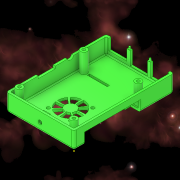
# Autodesk Inventor part: Bodem
Saved by Autodesk Inventor 2017 (Build 210142000, 142)
## iProperties
Created: 2016-12-17
Part Number: Bodem
Material: ABS Plastic
Document SubType Name: Modeling
Designer: bartv
Density: 1.06 g/cm^3
Appearance: Smooth - White
Author: bartv
## iProperties of the stored document Deksel_3DPrint.ipt
Created: 2016-12-19
Part Number: Deksel_3DPrint
Material: Generic
Document SubType Name: Modeling
Designer: bartv
Density: 1 g/cm^3
Appearance: Default
Author: bartv
Autodesk Inventor part; units mm, degrees
ref_plane "YZ Plane" through (0, 0, 0) normal (1, 0, 0) x (0, 1, 0)
ref_plane "XZ Plane" through (0, 0, 0) normal (0, 1, 0) x (-1, 0, 0)
ref_plane "XY Plane" through (0, 0, 0) normal (0, 0, 1) x (1, 0, 0)
sketch "Sketch3" plane through (0, 0, 0) normal (0, 1, 0) x (-1, 0, 0)
  line L0 (0, 0) -> (61, 0)
  line L1 (61, 0) -> (61, -90)
  line L2 (61, -90) -> (0, -90)
  line L3 (0, -90) -> (0, 0)
  dimension "d30" = 61
  dimension "d31" = 90
  constraints: 8 end point, 2 parallel, 1 horizontal, 1 perpendicular
  measures "d30" distance of L1.end L2.end
  measures "d31" distance between parallel lines of L0 L2
extrude "Extrusion2" add sketch "Sketch3" along normal blind 15.5
shell "Shell1" thickness 2 removed faces 1 at (-40.6667, 15.5, -60)
fillet "Fillet1" radius 2 8 edges at (-61, 7.75, 0) (0, 7.75, 0) (0, 7.75, -90) (-61, 7.75, -90) (-30.5, 0, -90) (-61, 0, -45) (-30.5, 0, 0) (0, 0, -45)
fillet "Fillet2" radius 1 8 edges at (-2, 2, -45) (-2, 8.75, -2) (-30.5, 2, -2) (-59, 2, -45) (-59, 8.75, -2) (-30.5, 2, -88) (-2, 8.75, -88) (-59, 8.75, -88)
sketch "Sketch4" plane through (-58, 2, -3) normal (0, 1, 0) x (1, 0, 0)
  circle A0 centre (52, 3) radius 1.375
  line L0 (-1, 0) -> (-1, 84) projected
  arc A1 (0, 85) -> (-1, 84) centre (0, 84) ccw projected
  line L1 (0, 85) -> (55, 85) projected
  arc A2 (56, 84) -> (55, 85) centre (55, 84) ccw projected
  line L2 (56, 84) -> (56, 0) projected
  arc A3 (55, -1) -> (56, 0) centre (55, 0) ccw projected
  line L3 (55, -1) -> (0, -1) projected
  arc A4 (-1, 0) -> (0, -1) centre (0, 0) ccw projected
  arc A5 (-3, -1) -> (-1, -3) centre (-1, -1) ccw projected
  line L4 (-1, -3) -> (56, -3) projected
  arc A6 (56, -3) -> (58, -1) centre (56, -1) ccw projected
  line L5 (58, -1) -> (58, 85) projected
  arc A7 (58, 85) -> (56, 87) centre (56, 85) ccw projected
  line L6 (56, 87) -> (-1, 87) projected
  arc A8 (-1, 87) -> (-3, 85) centre (-1, 85) ccw projected
  line L7 (-3, 85) -> (-3, -1) projected
  circle A9 centre (52, 61) radius 1.375
  circle A10 centre (3, 3) radius 1.375
  circle A11 centre (3, 61) radius 1.375
  circle A12 centre (52, 3) radius 3
  circle A13 centre (52, 61) radius 3
  circle A14 centre (3, 3) radius 3
  circle A15 centre (3, 61) radius 3
  point P0 (58, -3)
  dimension "d37" = 2.75
  dimension "d40" = 58
  dimension "d43" = 49
  dimension "d46" = 4
  dimension "d47" = 4
  dimension "d48" = 6
  dimension "d51" = 58
  dimension "d54" = 49
  constraints: 8 centre point, 4 coincident, 2 horizontal, 2 vertical, 15 other
  measures "d37" diameter of A0
  measures "d40" distance of A0.centre A9.centre
  measures "d43" distance of A0.centre A10.centre
  measures "d46" distance from line of L2 A0.centre
  measures "d47" distance from line of A0.centre L3
  measures "d48" diameter of A12
  measures "d51" distance of A0.centre point (52, 61)
  measures "d54" distance of A0.centre point (3, 3)
extrude "Extrusion3" add sketch "Sketch4" along normal blind 17.436 contours A12 | A13 | A14 | A15
sketch "Sketch5" plane through (-2, 15.5, -90) normal (0, 0, -1) x (-1, 0, 0)
  line L0 (54.6, -9.8) -> (38.2, -9.8)
  line L1 (38.2, -9.8) -> (38.2, 4.2)
  line L2 (38.2, 4.2) -> (54.6, 4.2)
  line L3 (54.6, 4.2) -> (54.6, -9.8)
  line L4 (57, 0) -> (57, -13.5) projected
  line L5 (0, 0) -> (57, 0) projected
  line L6 (35.3, -12) -> (19.8, -12)
  line L7 (19.8, -12) -> (19.8, 4.2)
  line L8 (19.8, 4.2) -> (35.3, 4.2)
  line L9 (35.3, 4.2) -> (35.3, -12)
  line L10 (16.9, -12) -> (1.4, -12)
  line L11 (1.4, -12) -> (1.4, 4.2)
  line L12 (1.4, 4.2) -> (16.9, 4.2)
  line L13 (16.9, 4.2) -> (16.9, -12)
  point P0 (-2, -15.5)
  dimension "d59" = 16.4
  dimension "d60" = 14
  dimension "d61" = 2.4
  dimension "d62" = 4.2
  dimension "d63" = 2.9
  dimension "d64" = 2.9
  dimension "d65" = 15.5
  dimension "d66" = 15.5
  dimension "d67" = 16.2
  dimension "d68" = 4.2
  constraints: 24 end point, 6 parallel, 3 horizontal, 3 perpendicular, 2 point on line
  measures "d59" distance between parallel lines of L1 L3
  measures "d60" distance of L0.end L1.end
  measures "d61" distance between parallel lines of L4 L3
  measures "d62" distance between parallel lines of L2 L5
  measures "d63" distance between parallel lines of L9 L1
  measures "d64" distance between parallel lines of L13 L7
  measures "d65" distance between parallel lines of L7 L9
  measures "d66" distance between parallel lines of L11 L13
  measures "d67" distance between parallel lines of L8 L6
  measures "d68" distance between parallel lines of L8 L5
extrude "Extrusion4" cut sketch "Sketch5" against normal up to surface (2 mm away)
sketch "Sketch7" plane through (-61, 2, -2) normal (-1, 0, 0) x (0, 0, 1)
  circle A0 centre (-54, 14.436) radius 3.05
  line L0 (-86, 13.5) -> (0, 13.5) projected
  line L1 (-88, 13.5) -> (-88, 0) projected
  line L2 (-40.1, 13.5) -> (-40.1, 11.356)
  line L3 (-40.1, 11.356) -> (-24.9, 11.356)
  line L4 (-24.9, 11.356) -> (-24.9, 13.5)
  line L5 (-24.9, 13.5) -> (-40.1, 13.5)
  point P0 (2, -2)
  dimension "d71" = 6.1
  dimension "d72" = 0.936
  dimension "d73" = 34
  dimension "d74" = 2.144
  dimension "d75" = 15.2
  dimension "d76" = 47.9
  constraints: 8 end point, 2 point on line, 1 centre point, 1 collinear, 1 perpendicular, 1 vertical
  measures "d71" diameter of A0
  measures "d72" distance from line of A0.centre L0
  measures "d73" distance from line of L1 A0.centre
  measures "d74" distance of L2.start L2.end
  measures "d75" distance of L2.end L3.end
  measures "d76" distance between parallel lines of L1 L2
extrude "Extrusion5" cut sketch "Sketch7" against normal up to surface (2 mm away)
sketch "Sketch11" plane through (-59, 2, 0) normal (0, 0, 1) x (1, 0, 0)
  point P0 (59, -2)
sketch "Sketch12" plane through (0, 0, 0) normal (0, -1, 0) x (1, 0, 0)
  circle A0 centre (-55, -6) radius 1.375 projected
  circle A1 centre (-55, -6) radius 2.5
  point P0 (0, 0)
  dimension "d85" = 5
  constraints: 1 centre point, 1 coincident
  measures "d85" diameter of A1
extrude "Extrusion7" cut sketch "Sketch12" against normal blind 16 contours A0 | A1
pattern_linear "Rectangular Pattern1" count 2 spacing 49 along (1, 0, 0) count 2 spacing 58 along (0, 0, -1) of "Extrusion7"
sketch "Sketch13" plane through (0, 0, 0) normal (0, -1, 0) x (1, 0, 0)
  line L0 (0, -9.5) -> (-10, -9.5)
  line L1 (-10, -9.5) -> (-10, -60)
  line L2 (-10, -60) -> (0, -60)
  line L3 (0, -60) -> (0, -9.5)
  line L4 (-2, -2) -> (-2, -88) projected
  line L5 (-59, -2) -> (-2, -2) projected
  circle A0 centre (-6, -6) radius 2.5 projected
  circle A1 centre (-6, -64) radius 3 projected
  line L6 (0, -88) -> (0, -2) projected
  line L7 (-61, -2) -> (-61, -88) projected
  point P0 (0, 0)
  point P1 (-3, -64)
  dimension "d100" = 3.5
  dimension "d101" = 1
  dimension "d102" = 0
  dimension "d103" = 51
  constraints: 8 end point, 2 parallel, 1 horizontal, 1 horizontal alignment, 1 perpendicular
  measures "d100" distance from line of L0 A0.centre
  measures "d102" distance between parallel lines of L6 L3
  measures "d103" distance between parallel lines of L1 L7
extrude "Extrusion8" cut sketch "Sketch13" against normal blind 10 contours L3 L2 L4 L0 | L4 L2 L1 L0
sketch "Sketch15" plane through (0, 0, 0) normal (0, -1, 0) x (1, 0, 0)
  line L0 (-51, -63) -> (-33, -63)
  line L1 (-33, -63) -> (-33, -65)
  line L2 (-33, -65) -> (-51, -65)
  line L3 (-51, -65) -> (-51, -63)
  line L4 (-61, -2) -> (-61, -88) projected
  line L5 (-56.6, -90) -> (-40.2, -90) projected
  point P0 (0, 0)
  dimension "d106" = 10
  dimension "d107" = 18
  dimension "d108" = 2
  dimension "d109" = 25
  constraints: 8 end point, 2 parallel, 1 horizontal, 1 perpendicular
  measures "d106" distance between parallel lines of L4 L3
  measures "d107" distance of L1.end L2.end
  measures "d108" distance between parallel lines of L0 L2
  measures "d109" distance between parallel lines of L5 L2
extrude "Extrusion9" cut sketch "Sketch15" against normal through all
sketch "Sketch16" plane through (0, 15.5, 0) normal (0, 1, 0) x (1, 0, 0)
  circle A0 centre (-38.8, 89) radius 0.75
  line L0 (-37.3, 88) -> (-37.3, 90) projected
  line L1 (-40.2, 88) -> (-37.3, 88) projected
  circle A1 centre (-20.4, 89) radius 0.75
  line L2 (-18.9, 88) -> (-18.9, 90) projected
  line L3 (-21.8, 88) -> (-18.9, 88) projected
  point P0 (0, 0)
  dimension "d113" = 1.5
  dimension "d114" = 1.5
  dimension "d115" = 1
  dimension "d116" = 1.5
  dimension "d117" = 1.5
  dimension "d118" = 1
  constraints: 2 centre point
  measures "d113" diameter of A0
  measures "d114" distance from line of L0 A0.centre
  measures "d115" distance from line of L1 A0.centre
  measures "d116" diameter of A1
  measures "d117" distance from line of L2 A1.centre
  measures "d118" distance from line of L3 A1.centre
extrude "Extrusion10" add sketch "Sketch16" along normal blind 2
sketch "Sketch17" plane through (0, 0, 0) normal (0, -1, 0) x (1, 0, 0)
  circle A0 centre (-23, -20) radius 1.5
  circle A1 centre (-43, -20) radius 1.5
  line L0 (-2, 0) -> (-59, 0) projected
  line L1 (-61, -2) -> (-61, -88) projected
  circle A2 centre (-23, -40) radius 1.5
  line L2 (-23, -40) -> (-23, -20) construction
  line L3 (-23, -20) -> (-43, -20) construction
  circle A3 centre (-33, -30) radius 11.75
  circle A4 centre (-33, -30) radius 5
  arc A5 (-28, -30) -> (-21.25, -30) centre (-24.625, -12.3192) ccw
  arc A6 (-28.101, -31) -> (-21.3887, -31.8) centre (-22.6525, -13.8444) ccw
  circle A7 centre (-33, -30) radius 5
  arc A8 (-29.4645, -26.4645) -> (-24.6915, -21.6915) centre (-39.5802, -11.5758) ccw
  arc A9 (-28.8288, -27.243) -> (-23.5168, -23.0624) centre (-37.1069, -11.2595) ccw
  circle A10 centre (-33, -30) radius 11.75
  circle A11 centre (-33, -30) radius 5
  arc A12 (-33, -25) -> (-33, -18.25) centre (-50.6808, -21.625) ccw
  arc A13 (-32, -25.101) -> (-31.2, -18.3887) centre (-49.1556, -19.6525) ccw
  circle A14 centre (-33, -30) radius 11.75
  circle A15 centre (-33, -30) radius 5
  arc A16 (-36.5355, -26.4645) -> (-41.3085, -21.6915) centre (-51.4242, -36.5802) ccw
  arc A17 (-35.757, -25.8288) -> (-39.9376, -20.5168) centre (-51.7405, -34.1069) ccw
  circle A18 centre (-33, -30) radius 11.75
  circle A19 centre (-33, -30) radius 5
  arc A20 (-38, -30) -> (-44.75, -30) centre (-41.375, -47.6808) ccw
  arc A21 (-37.899, -29) -> (-44.6113, -28.2) centre (-43.3475, -46.1556) ccw
  circle A22 centre (-33, -30) radius 11.75
  circle A23 centre (-33, -30) radius 5
  arc A24 (-36.5355, -33.5355) -> (-41.3085, -38.3085) centre (-26.4198, -48.4242) ccw
  arc A25 (-37.1712, -32.757) -> (-42.4832, -36.9376) centre (-28.8931, -48.7405) ccw
  circle A26 centre (-33, -30) radius 11.75
  circle A27 centre (-33, -30) radius 5
  arc A28 (-33, -35) -> (-33, -41.75) centre (-15.3192, -38.375) ccw
  arc A29 (-34, -34.899) -> (-34.8, -41.6113) centre (-16.8444, -40.3475) ccw
  circle A30 centre (-33, -30) radius 11.75
  circle A31 centre (-33, -30) radius 5
  arc A32 (-29.4645, -33.5355) -> (-24.6915, -38.3085) centre (-14.5758, -23.4198) ccw
  arc A33 (-30.243, -34.1712) -> (-26.0624, -39.4832) centre (-14.2595, -25.8931) ccw
  circle A34 centre (-33, -30) radius 11.75
  point P0 (0, 0)
  dimension "d121" = 3
  dimension "d122" = 3
  dimension "d123" = 20
  dimension "d124" = 20
  dimension "d125" = 18
  dimension "d126" = 3
  dimension "d144" = 23.5
  dimension "d145" = 10
  dimension "d146" = 18
  dimension "d147" = 18
  dimension "d148" = 10
  dimension "d149" = 10
  dimension "d150" = 1
  dimension "d151" = 1.8
  dimension "d154" = 360
  constraints: 64 point on circle, 35 centre point, 10 coincident, 4 end point, 1 perpendicular, 1 vertical, 95 other
  measures "d121" diameter of A0
  measures "d122" diameter of A1
  measures "d123" distance of L3.end L2.end
  measures "d124" distance from line of L0 L2.end
  measures "d125" distance from line of L1 L3.end
  measures "d126" diameter of A2
  measures "d144" diameter of A3
  measures "d145" diameter of A4
  measures "d146" radius of A5
  measures "d147" radius of A6
  measures "d148" distance from line of L2 A3.centre
  measures "d149" distance from line of L3 A3.centre
  measures "d150" vertical distance of A4.end A4.start
  measures "d151" vertical distance of A3.start A3.end
extrude "Extrusion11" cut sketch "Sketch17" against normal blind 2 contours A0 | A1 | A2 | A5 A4 A9 A3 | A3 A32 A4 A6 | A8 A4 A13 A3 | A3 A28 A4 A33 | A12 A4 A17 A3 | A3 A24 A4 A29 | A16 A4 A21 A3 | A3 A20 A4 A25
sketch "Sketch18" plane through (-3, 3, -2) normal (0, 0, -1) x (-1, 0, 0)
  line L0 (30.525, 1) -> (24.475, 1)
  line L1 (24.475, 1) -> (24.475, 7.05)
  line L2 (24.475, 7.05) -> (30.525, 7.05)
  line L3 (30.525, 7.05) -> (30.525, 1)
  line L4 (55, 0) -> (0, 0) projected
  line L5 (55, 12.5) -> (55, 0) projected
  point P0 (-3, -3)
  dimension "d156" = 6.05
  dimension "d157" = 6.05
  dimension "d158" = 1
  dimension "d159" = 24.475
  constraints: 8 end point, 2 parallel, 1 horizontal, 1 perpendicular
  measures "d156" distance of L1.end L2.end
  measures "d157" distance between parallel lines of L2 L0
  measures "d158" distance between parallel lines of L0 L4
  measures "d159" distance between parallel lines of L5 L3
extrude "Extrusion12" cut sketch "Sketch18" against normal blind 1
sketch "Sketch19" plane through (-3, 3, -1) normal (0, 0, -1) x (-1, 0, 0)
  line L0 (30.525, 1) -> (24.475, 1) construction
  line L1 (30.525, 7.05) -> (30.525, 1) construction
  line L2 (24.475, 7.05) -> (30.525, 7.05) construction
  line L3 (24.475, 1) -> (24.475, 7.05) construction
  line L4 (30.525, 1) -> (24.475, 7.05) construction
  line L5 (24.475, 1) -> (30.525, 7.05) construction
  circle A0 centre (27.5, 4.025) radius 1.75
  point P0 (-3, -3)
  dimension "d162" = 3.5
  constraints: 4 end point, 1 centre point, 1 midpoint, 1 perpendicular
  measures "d162" diameter of A0
extrude "Extrusion13" cut sketch "Sketch19" against normal blind 1
sketch "Sketch21" plane through (-58, 2, -87) normal (0, 1, 0) x (1, 0, 0)
  line L0 (24.475, -80.85) -> (30.525, -80.85)
  line L1 (30.525, -80.85) -> (30.525, -82.35)
  line L2 (30.525, -82.35) -> (24.475, -82.35)
  line L3 (24.475, -82.35) -> (24.475, -80.85)
  line L4 (55, -85) -> (0, -85) projected
  line L5 (24.475, -85) -> (24.475, -86) projected
  line L6 (30.525, -85) -> (30.525, -86) projected
  point P0 (58, -87)
  dimension "d165" = 2.65
  dimension "d166" = 1.5
  constraints: 8 end point, 2 collinear, 2 parallel, 1 horizontal, 1 perpendicular
  measures "d165" distance between parallel lines of L4 L2
  measures "d166" distance between parallel lines of L2 L0
extrude "Extrusion14" add sketch "Sketch21" along normal blind 10
sketch "Sketch22" plane through (0, 10, 0) normal (0, -1, 0) x (1, 0, 0)
  line L0 (-2, -60) -> (-1, -60)
  line L1 (-1, -60) -> (-1, -55)
  line L2 (-1, -55) -> (-2, -55)
  line L3 (-2, -55) -> (-2, -60)
  line L4 (-2, -9.4618) -> (-1, -9.4618)
  line L5 (-1, -9.4618) -> (-1, -14.5)
  line L6 (-1, -14.5) -> (-2, -14.5)
  line L7 (-2, -14.5) -> (-2, -9.4618)
  line L8 (-2, -60) -> (-2, -9.5) projected
  line L9 (0, -60) -> (-2, -60) projected
  line L10 (0, -9.5) -> (0, -60) projected
  line L11 (-2, -9.5) -> (0, -9.5) projected
  point P0 (0, 0)
  dimension "d169" = 1
  dimension "d170" = 5
  dimension "d171" = 1
  dimension "d172" = 5
  dimension "d173" = 1
  dimension "d174" = 5
  constraints: 16 end point, 4 parallel, 2 horizontal, 2 perpendicular, 1 point on line
  measures "d169" distance between parallel lines of L1 L3
  measures "d170" distance between parallel lines of L2 L0
  measures "d171" distance between parallel lines of L10 L1
  measures "d172" distance between parallel lines of L11 L6
  measures "d173" distance between parallel lines of L10 L5
  measures "d174" distance between parallel lines of L9 L2
extrude "Extrusion15" cut sketch "Sketch22" against normal blind 2 contours L3 L2 L1 L0 | L7 L11 L5 L6 | L7 L4 L5 L11
sketch "Sketch23" plane through (-10, 0, -9.5) normal (1, 0, 0) x (0, 0, -1)
  line L0 (0, 2) -> (50.5, 2) projected
  line L1 (0, 0) -> (0, 2) projected
  line L2 (50.5, 0) -> (0, 0) projected
  line L3 (50.5, 0) -> (50.5, 2) projected
  line L4 (50.5, 0) -> (45.5, 0)
  line L5 (45.5, 0) -> (45.5, 1)
  line L6 (45.5, 1) -> (50.5, 1)
  line L7 (50.5, 1) -> (50.5, 0)
  line L8 (0, 0) -> (5, 0)
  line L9 (5, 0) -> (5, 1)
  line L10 (5, 1) -> (0, 1)
  line L11 (0, 1) -> (0, 0)
  point P0 (-9.5, 0)
  dimension "d177" = 5
  dimension "d178" = 5
  dimension "d179" = 1
  constraints: 16 end point, 4 parallel, 2 horizontal, 2 perpendicular, 1 point on line
  measures "d177" distance of L5.end L6.end
  measures "d178" distance of L10.end L9.end
  measures "d179" distance between parallel lines of L0 L10
extrude "Extrusion16" add sketch "Sketch23" along normal blind 1 contours L10 L9 L2 L1 | L3 L2 L5 L6
body "Solid2"
